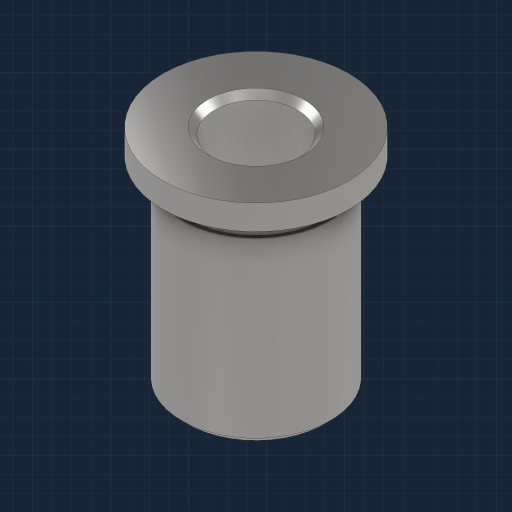
# Autodesk Inventor part: s14-13
Saved by Autodesk Inventor 2024 (Build 280153000, 153)
## iProperties
Created: 2026-04-25
Part Number: s14-13
Material: Steel, Carbon
Document SubType Name: Modeling
Designer: DuctopwH
Density: 7.85 g/cm^3
Appearance: Semi-Polished
Author: DuctopwH
Autodesk Inventor part; units mm, degrees
ref_plane "YZ Plane" through (0, 0, 0) normal (1, 0, 0) x (0, 1, 0)
ref_plane "XZ Plane" through (0, 0, 0) normal (0, 1, 0) x (-1, 0, 0)
ref_plane "XY Plane" through (0, 0, 0) normal (0, 0, 1) x (1, 0, 0)
sketch "Sketch1" plane through (0, 0, 0) normal (0, 0, 1) x (1, 0, 0)
  line L0 (0, 0) -> (0, 18)
  line L1 (0, 0) -> (-6, 0)
  line L2 (-6, 0) -> (-6, 16)
  line L3 (-6, 16) -> (-7.5, 16)
  line L4 (-7.5, 16) -> (-7.5, 18)
  line L5 (-7.5, 18) -> (0, 18)
  dimension "d0" = 18
  dimension "d1" = 15
  dimension "d2" = 12
  dimension "d3" = 2
  constraints: 12 end point, 4 perpendicular, 1 horizontal, 1 vertical
  measures "d0" distance between parallel lines of L1 L5
  measures "d1" diameter of L4 L0
  measures "d2" diameter of L2 L0
  measures "d3" distance of L3.end L4.end
revolve "Revolution1" add sketch "Sketch1" angle 360 about axis through (0, 0, 0) along (0, 1, 0)
sketch "Sketch2" plane through (0, 0, 0) normal (0, 0, 1) x (1, 0, 0)
  line L0 (7.5, 16) -> (-7.5, 16) projected
  line L1 (-6, 0) -> (-6, 16) projected
  line L2 (-6, 14.5) -> (-5.75, 14.5)
  line L3 (-5.75, 14.5) -> (-5.75, 16)
  line L4 (0, 16) -> (0, 9.2067)
  point P0 (0, 0)
  dimension "d5" = 11.5
  dimension "d6" = 1.5
  constraints: 6 end point, 2 point on line, 1 horizontal, 1 midpoint, 1 perpendicular, 1 vertical
  measures "d5" diameter of L3 L4
  measures "d6" distance of L2.end L3.end
revolve "Revolution2" cut sketch "Sketch2" angle 360 about axis through (0, 16, 0) along (0, -1, 0)
sketch "Sketch3" plane through (0, 18, 0) normal (0, 1, 0) x (1, 0, 0)
  circle A0 centre (0, 0) radius 7.5 projected
  constraints: 1 coincident
hole "d6.75" at (0, 18, 0) direction (0, -1, 0) diameter 6.75 end through all
chamfer "0.5x45" distance 0.5 angle 45 2 edges at (0, 18, -3.375) (6, 0, 0)
body "Solid1"
